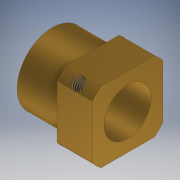
# Autodesk Inventor part: TH81-RS81
Saved by Autodesk Inventor 2017.1 (Build 211199000, 199)
## iProperties
Category: Bag #1
Company: Autodesk Inc.
Created: 2016-12-26
Part Number: TH81-RS81
Material: Aluminum 6061
Document SubType Name: Modeling
Designer: Autodesk Inc.
Density: 2.7 g/cm^3
Appearance: Brass - Satin
Catalog Web Link: www.banebots.com
Vendor: BaneBots
Author: Autodesk Inc.
Keywords: Gray Tote
Autodesk Inventor part; units mm, degrees
ref_plane "YZ Plane" through (0, 0, 0) normal (1, 0, 0) x (0, 1, 0)
ref_plane "XZ Plane" through (0, 0, 0) normal (0, 1, 0) x (-1, 0, 0)
sketch "Sketch1" plane through (0, 0, 0) normal (0, 1, 0) x (-1, 0, 0)
  circle A0 centre (0, 0) radius 6.35
  line L0 (9.525, 7.1772) -> (9.525, -7.1772)
  line L1 (-9.525, 7.1772) -> (-9.525, -7.1772)
  line L2 (7.1772, 9.525) -> (-7.1772, 9.525)
  line L3 (7.1772, -9.525) -> (-7.1772, -9.525)
  arc A1 (7.1772, -9.525) -> (9.525, -7.1772) centre (0, 0) ccw
  arc A2 (9.525, 7.1772) -> (7.1772, 9.525) centre (0, 0) ccw
  arc A3 (-7.1772, 9.525) -> (-9.525, 7.1772) centre (0, 0) ccw
  arc A4 (-9.525, -7.1772) -> (-7.1772, -9.525) centre (0, 0) ccw
  dimension "d0" = 12.7
  dimension "d2" = 9.525
  dimension "d3" = 9.525
  dimension "d4" = 9.525
  dimension "d5" = 9.525
  constraints: 8 end point, 8 point on circle, 5 centre point, 3 coincident, 2 horizontal, 2 vertical
  measures "d0" diameter of A0
  measures "d2" distance from line of point (0, 0) L0
  measures "d3" distance from line of L1 point (0, 0)
  measures "d4" distance from line of L2 point (0, 0)
  measures "d5" distance from line of L3 point (0, 0)
extrude "Extrusion1" add sketch "Sketch1" against normal blind 9.525
sketch "Sketch2" plane through (0, -9.525, 0) normal (0, -1, 0) x (1, 0, 0)
  circle A0 centre (0, 0) radius 9.525
  circle A1 centre (0, 0) radius 6.35 projected
  dimension "d8" = 19.05
  constraints: 1 centre point, 1 coincident
  measures "d8" diameter of A0
extrude "Extrusion2" add sketch "Sketch2" along normal blind 10.795
ref_plane "Work Plane2" through (-15.1377, 0, -12.7898) normal (0.7071068, 0, 0.7071068) x (0, -1, 0)
ref_plane "Work Plane1" through (-9.525, 0, -7.1772) normal (0.7071068, 0, 0.7071068) x (0, -1, 0)
sketch "Sketch3" plane through (-15.1377, 0, -12.7898) normal (0.7071068, 0, 0.7071068) x (0, -1, 0)
  line L0 (0, 3.3203) -> (9.525, 3.3203) projected
  line L1 (0, 0) -> (9.525, 0) projected
  point P0 (0, 1.6602)
  point P1 (4.7625, 1.6602)
hole "Hole1" at (-13.9638, -4.7625, -13.9638) direction (0.7071068, 0, 0.7071068) diameter 3.302 end up to surface thread size "8-32 UNC" class "2B" standard "ANSI Unified Screw Threads"
equation "\"d3\" = d2"
equation "\"d4\" = d2"
equation "\"d5\" = d4"
body "Solid1"
